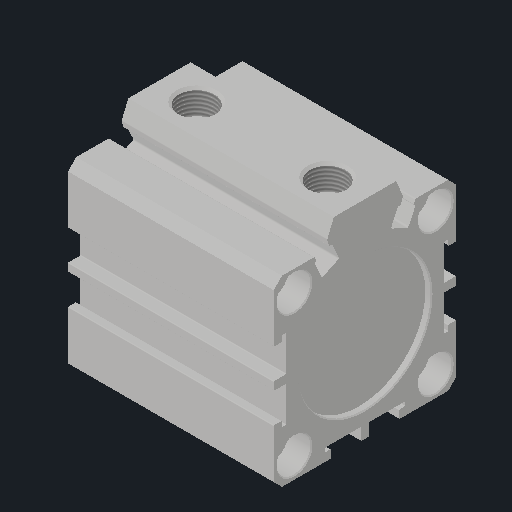
# Autodesk Inventor part: SDA-32x2525_b
Saved by Autodesk Inventor 2022 (Build 260153000, 153)
## iProperties
Created: 2022-09-20
Part Number: SDA-32x2525_b
Material: Generic
Catalog Web Link: www.cadenas.de
Description: SDA SSA STA  Series - Body-Body
Vendor: AIRTAC
Document SubType Name: Modeling
Designer: psAdmin
Manufacturer: AIRTAC
Mass: 56.8028 g
Surface Area: 257.905 cm^2
Volume: 56.8028 cm^3
Density: 1 g/cm^3
Appearance: PSOLRGB-175-175-175
Category: PARTsolutions
Company: AIRTAC
PSOL_IDENT_0: {$CADENAS_DATA/23d-libs/airtac/pneumatic_equipment/cylinders/compact_cylinder/sda_series/parts/sda_s
PSOL_IDENT_1: sa_sta_body.prj},222 {VTYP=3D},{NB=SDA-32x2525_b},{LINA=SDA-32x25},{NN=SDA SSA STA  Series - Body},{
PSOL_IDENT_2: DATE=27.08.2021 03:42:34},{GEOMDATE=22.01.2019 02:43:44},{VERSION=},{LINEID=50},{WBVAR=TYPE,STROKE,S
PSOL_IDENT_3: TROKE1,MAGNET},{WBNUMERIC=STROKE,STROKE1}  {NB=SDA-32x2525_b},{LINA=SDA-32x25},{KT=DUMMY},{BORE=32},
PSOL_IDENT_4: {TYPE=SDA},{STROKE=25},{STROKE1=25},{MAGNET=},{ST1=5,10,15,20,25,30,35,40,45,50,55,60,65,70,75,80,85
PSOL_IDENT_5: ,90,100,110,120,130,[5:100]},{ORDER=SDA-32x25},{A=31.5},{B1=7.0},{C=24.5},{D=50.0},{E=12},{F=4},{G=3
PSOL_IDENT_6: .0},{K1=M6×1.0},{L=22.0},{M=3},{N1=9.0},{N2=9.0},{O=PT1/8},{P1=4.6},{P2=M6×1.0},{P3=16},{P4=5.5},{P5=
PSOL_IDENT_7: 8.2},{R=6},{S=44.000},{T1=34.0},{U=2.0},{V=12},{W=10},{X=18.3},{Y=15},{TYPE1='SDA', 'SDA Type', 'SSA'
PSOL_IDENT_8: , 'SSA Type', 'STA', 'STA Type'},{X1=40.5},{ST2=25}
NB: SDA-32x2525_b
NN: SDA SSA STA  Series - Body
NT: Body
NBSYN: $ORDER.$STROKE._b
LINA: SDA-32x25
CATALOG: AirTAC
BORE: 32
TYPE: SDA Type
STROKE: 25
STROKE1: 25
MAGNET: Without cushion
A: 31.5
B1: 7
C: 24.5
D: 50
E: 12
F: 4
G: 3
K1: M6×1.0
L: 22
M: 3
N1: 9
N2: 9
O: PT1/8
P1: 4.6
P2: M6×1.0
P3: 16
P4: 5.5
P5: 8.2
R: 6
S: 44
T1: 34
U: 2
V: 12
W: 10
X: 18.3
Y: 15
SUPPLIER: AIRTAC
ARTICLENO: SDA-32x2525_b
BOMINFO: SDA-32x25
CREATOR: CADENAS GmbH
Title: SDA-32x25
Author: Cadenas PARTsolutions
Comments: Body
Autodesk Inventor part; units mm, degrees
sketch "Sketch_1" plane through (0, 0, 0) normal (1, 0, 0) x (0, 1, 0)
  line L0 (0.8, 22) -> (-0.8, 22)
  arc A0 (-0.8, 22) -> (-1, 21.8) centre (-0.8, 21.8) ccw
  line L1 (-1, 21.8) -> (-1, 19.2)
  arc A1 (-1.2, 19) -> (-1, 19.2) centre (-1.2, 19.2) ccw
  line L2 (-1.2, 19) -> (-9.4, 19)
  arc A2 (-9.6, 19.2) -> (-9.4, 19) centre (-9.4, 19.2) ccw
  line L3 (-9.6, 19.2) -> (-9.6, 19.8)
  arc A3 (-9.4, 20) -> (-9.6, 19.8) centre (-9.4, 19.8) ccw
  line L4 (-9.4, 20) -> (-8.4, 20)
  arc A4 (-8.4, 20) -> (-8.2, 20.2) centre (-8.4, 20.2) ccw
  line L5 (-8.2, 20.2) -> (-8.2, 21.8)
  arc A5 (-8.2, 21.8) -> (-8.4, 22) centre (-8.4, 21.8) ccw
  line L6 (-8.4, 22) -> (-20, 22)
  line L7 (-20, 22) -> (-22, 20)
  line L8 (-22, 20) -> (-22, 8.4)
  arc A6 (-22, 8.4) -> (-21.8, 8.2) centre (-21.8, 8.4) ccw
  line L9 (-21.8, 8.2) -> (-20.2, 8.2)
  arc A7 (-20.2, 8.2) -> (-20, 8.4) centre (-20.2, 8.4) ccw
  line L10 (-20, 8.4) -> (-20, 9.4)
  arc A8 (-19.8, 9.6) -> (-20, 9.4) centre (-19.8, 9.4) ccw
  line L11 (-19.8, 9.6) -> (-19.2, 9.6)
  arc A9 (-19, 9.4) -> (-19.2, 9.6) centre (-19.2, 9.4) ccw
  line L12 (-19, 9.4) -> (-19, 1.2)
  arc A10 (-19.2, 1) -> (-19, 1.2) centre (-19.2, 1.2) ccw
  line L13 (-19.2, 1) -> (-21.8, 1)
  arc A11 (-21.8, 1) -> (-22, 0.8) centre (-21.8, 0.8) ccw
  line L14 (-22, 0.8) -> (-22, -0.8)
  arc A12 (-22, -0.8) -> (-21.8, -1) centre (-21.8, -0.8) ccw
  line L15 (-21.8, -1) -> (-19.2, -1)
  arc A13 (-19, -1.2) -> (-19.2, -1) centre (-19.2, -1.2) ccw
  line L16 (-19, -1.2) -> (-19, -9.4)
  arc A14 (-19.2, -9.6) -> (-19, -9.4) centre (-19.2, -9.4) ccw
  line L17 (-19.2, -9.6) -> (-19.8, -9.6)
  arc A15 (-20, -9.4) -> (-19.8, -9.6) centre (-19.8, -9.4) ccw
  line L18 (-20, -9.4) -> (-20, -8.4)
  arc A16 (-20, -8.4) -> (-20.2, -8.2) centre (-20.2, -8.4) ccw
  line L19 (-20.2, -8.2) -> (-21.8, -8.2)
  arc A17 (-21.8, -8.2) -> (-22, -8.4) centre (-21.8, -8.4) ccw
  line L20 (-22, -8.4) -> (-22, -20)
  line L21 (-22, -20) -> (-20, -22)
  line L22 (-20, -22) -> (-8.4, -22)
  arc A18 (-8.4, -22) -> (-8.2, -21.8) centre (-8.4, -21.8) ccw
  line L23 (-8.2, -21.8) -> (-8.2, -20.2)
  arc A19 (-8.2, -20.2) -> (-8.4, -20) centre (-8.4, -20.2) ccw
  line L24 (-8.4, -20) -> (-9.4, -20)
  arc A20 (-9.6, -19.8) -> (-9.4, -20) centre (-9.4, -19.8) ccw
  line L25 (-9.6, -19.8) -> (-9.6, -19.2)
  arc A21 (-9.4, -19) -> (-9.6, -19.2) centre (-9.4, -19.2) ccw
  line L26 (-9.4, -19) -> (-1.2, -19)
  arc A22 (-1, -19.2) -> (-1.2, -19) centre (-1.2, -19.2) ccw
  line L27 (-1, -19.2) -> (-1, -21.8)
  arc A23 (-1, -21.8) -> (-0.8, -22) centre (-0.8, -21.8) ccw
  line L28 (-0.8, -22) -> (0.8, -22)
  arc A24 (0.8, -22) -> (1, -21.8) centre (0.8, -21.8) ccw
  line L29 (1, -21.8) -> (1, -19.2)
  arc A25 (1.2, -19) -> (1, -19.2) centre (1.2, -19.2) ccw
  line L30 (1.2, -19) -> (9.4, -19)
  arc A26 (9.6, -19.2) -> (9.4, -19) centre (9.4, -19.2) ccw
  line L31 (9.6, -19.2) -> (9.6, -19.8)
  arc A27 (9.4, -20) -> (9.6, -19.8) centre (9.4, -19.8) ccw
  line L32 (9.4, -20) -> (8.4, -20)
  arc A28 (8.4, -20) -> (8.2, -20.2) centre (8.4, -20.2) ccw
  line L33 (8.2, -20.2) -> (8.2, -21.8)
  arc A29 (8.2, -21.8) -> (8.4, -22) centre (8.4, -21.8) ccw
  line L34 (8.4, -22) -> (20, -22)
  line L35 (20, -22) -> (22, -20)
  line L36 (22, -20) -> (22, -12.3893)
  arc A30 (22, -12.3893) -> (21.769, -12.0268) centre (21.6, -12.3893) ccw
  line L37 (21.769, -12.0268) -> (21.1236, -11.7258)
  arc A31 (21.1236, -11.7258) -> (20.8578, -11.8226) centre (21.039, -11.9071) ccw
  line L38 (20.8578, -11.8226) -> (20.7733, -12.0038)
  arc A32 (20.5075, -12.1006) -> (20.7733, -12.0038) centre (20.592, -11.9193) ccw
  line L39 (20.5075, -12.1006) -> (17.1541, -10.5369)
  arc A33 (16.9607, -10.0053) -> (17.1541, -10.5369) centre (17.3232, -10.1744) ccw
  line L40 (16.9607, -10.0053) -> (18.5666, -6.5613)
  arc A34 (19.0982, -6.3679) -> (18.5666, -6.5613) centre (18.9291, -6.7304) ccw
  line L41 (19.0982, -6.3679) -> (22.4515, -7.9315)
  arc A35 (22.5483, -8.1973) -> (22.4515, -7.9315) centre (22.367, -8.1128) ccw
  line L42 (22.5483, -8.1973) -> (22.4749, -8.3546)
  arc A36 (22.4749, -8.3546) -> (22.5947, -8.6294) centre (22.6562, -8.4391) ccw
  line L43 (22.5947, -8.6294) -> (23.96, -9.0702)
  arc A37 (23.96, -9.0702) -> (24.2359, -9.0591) centre (24.0829, -8.6896) ccw
  line L44 (24.2359, -9.0591) -> (28, -7.5)
  line L45 (28, -7.5) -> (28, 7.5)
  line L46 (28, 7.5) -> (24.2359, 9.0591)
  arc A38 (24.2359, 9.0591) -> (23.96, 9.0702) centre (24.0829, 8.6896) ccw
  line L47 (23.96, 9.0702) -> (22.5947, 8.6294)
  arc A39 (22.5947, 8.6294) -> (22.4749, 8.3546) centre (22.6562, 8.4391) ccw
  line L48 (22.4749, 8.3546) -> (22.5483, 8.1973)
  arc A40 (22.4515, 7.9315) -> (22.5483, 8.1973) centre (22.367, 8.1128) ccw
  line L49 (22.4515, 7.9315) -> (19.0982, 6.3679)
  arc A41 (18.5666, 6.5613) -> (19.0982, 6.3679) centre (18.9291, 6.7304) ccw
  line L50 (18.5666, 6.5613) -> (16.9607, 10.0053)
  arc A42 (17.1541, 10.5369) -> (16.9607, 10.0053) centre (17.3232, 10.1744) ccw
  line L51 (17.1541, 10.5369) -> (20.5075, 12.1006)
  arc A43 (20.7733, 12.0038) -> (20.5075, 12.1006) centre (20.592, 11.9193) ccw
  line L52 (20.7733, 12.0038) -> (20.8578, 11.8226)
  arc A44 (20.8578, 11.8226) -> (21.1236, 11.7258) centre (21.039, 11.9071) ccw
  line L53 (21.1236, 11.7258) -> (21.769, 12.0268)
  arc A45 (21.769, 12.0268) -> (22, 12.3893) centre (21.6, 12.3893) ccw
  line L54 (22, 12.3893) -> (22, 20)
  line L55 (22, 20) -> (20, 22)
  line L56 (20, 22) -> (8.4, 22)
  arc A46 (8.4, 22) -> (8.2, 21.8) centre (8.4, 21.8) ccw
  line L57 (8.2, 21.8) -> (8.2, 20.2)
  arc A47 (8.2, 20.2) -> (8.4, 20) centre (8.4, 20.2) ccw
  line L58 (8.4, 20) -> (9.4, 20)
  arc A48 (9.6, 19.8) -> (9.4, 20) centre (9.4, 19.8) ccw
  line L59 (9.6, 19.8) -> (9.6, 19.2)
  arc A49 (9.4, 19) -> (9.6, 19.2) centre (9.4, 19.2) ccw
  line L60 (9.4, 19) -> (1.2, 19)
  arc A50 (1, 19.2) -> (1.2, 19) centre (1.2, 19.2) ccw
  line L61 (1, 19.2) -> (1, 21.8)
  arc A51 (1, 21.8) -> (0.8, 22) centre (0.8, 21.8) ccw
  constraints: 124 end point, 104 point on circle, 52 centre point
extrude "Extrusion1" add sketch "Sketch_1" along normal blind 49.5
sketch "Sketch_4" plane through (0, 0, 17) normal (0, 0, 1) x (1, 0, 0)
  line L0 (24.75, -17) -> (0, -17)
  line L1 (0, -17) -> (0, -12.65)
  line L2 (0, -12.65) -> (0.25, -12.9)
  line L3 (0.25, -12.9) -> (5.5, -12.9)
  line L4 (5.5, -12.9) -> (5.5, -14)
  line L5 (5.5, -14) -> (6.0415, -14.5415)
  line L6 (6.0415, -14.5415) -> (15.4585, -14.5415)
  line L7 (15.4585, -14.5415) -> (16, -14)
  line L8 (16, -14) -> (16, -14.7)
  line L9 (16, -14.7) -> (24.75, -14.7)
  line L10 (24.75, -14.7) -> (24.75, -17)
  line L11 (24.75, -17) -> (0, -17)
  constraints: 24 end point
revolve "Revolution1" cut sketch "Sketch_4" angle 360 about axis through (24.75, -17, 17) along (1, 0, 0)
thread "Thread1" size "M6x1" class "6H" standard "ISO Metric profile" full length
pattern_linear "Rectangular Pattern1" count 2 spacing 34 along (0, 0, -1) count 2 spacing 34 along (0, 1, 0) of "Revolution1"
sketch "Sketch_5" plane through (0, 0, 17) normal (0, 0, 1) x (1, 0, 0)
  line L0 (49.5, -17) -> (24.75, -17)
  line L1 (24.75, -17) -> (24.75, -14.7)
  line L2 (24.75, -14.7) -> (33.5, -14.7)
  line L3 (33.5, -14.7) -> (33.5, -14)
  line L4 (33.5, -14) -> (34.0415, -14.5415)
  line L5 (34.0415, -14.5415) -> (43.4585, -14.5415)
  line L6 (43.4585, -14.5415) -> (44, -14)
  line L7 (44, -14) -> (44, -12.9)
  line L8 (44, -12.9) -> (49.25, -12.9)
  line L9 (49.25, -12.9) -> (49.5, -12.65)
  line L10 (49.5, -12.65) -> (49.5, -17)
  line L11 (49.5, -17) -> (24.75, -17)
  constraints: 24 end point
revolve "Revolution2" cut sketch "Sketch_5" angle 360 about axis through (49.5, -17, 17) along (1, 0, 0)
thread "Thread2" size "M6x1" class "6H" standard "ISO Metric profile" full length
pattern_linear "Rectangular Pattern2" count 2 spacing 34 along (0, 0, -1) count 2 spacing 34 along (0, 1, 0) of "Revolution2"
sketch "Sketch4" plane through (0, 28, 7.5) normal (0, 1, 0) x (1, 0, 0)
  point P0 (9, 7.5)
hole "Hole1" at (9, 28, 0) direction (0, -1, 0) diameter 8.566 depth 6 countersink diameter 9.728 countersink angle 90 thread size "G9.728x0.907" designation "G 1/8" standard "ISO Pipe Threads"
sketch "Sketch5" plane through (0, 28, 7.5) normal (0, 1, 0) x (1, 0, 0)
  point P0 (40.5, 7.5)
hole "Hole2" at (40.5, 28, 0) direction (0, -1, 0) diameter 8.566 depth 6 countersink diameter 9.728 countersink angle 90 thread size "G9.728x0.907" designation "G 1/8" standard "ISO Pipe Threads"
sketch "Sketch_10" plane through (0, 0, 0) normal (0, 0, 1) x (1, 0, 0)
  line L0 (43.5, 0) -> (0, 0)
  line L1 (0, 0) -> (0, 6)
  line L2 (0, 6) -> (11.3, 6)
  line L3 (11.3, 6) -> (11.3, 16)
  line L4 (11.3, 16) -> (43.5, 16)
  line L5 (43.5, 16) -> (43.5, 0)
  line L6 (43.5, 0) -> (0, 0)
  constraints: 14 end point
revolve "Revolution3" cut sketch "Sketch_10" angle 360 about axis through (43.5, 0, 0) along (1, 0, 0)
sketch "Sketch_11" plane through (0, 0, 0) normal (0, 0, 1) x (1, 0, 0)
  line L0 (2.5, 0) -> (0, 0)
  line L1 (0, 0) -> (0, 17.4)
  line L2 (0, 17.4) -> (0.4, 17)
  line L3 (0.4, 17) -> (2.5, 17)
  line L4 (2.5, 17) -> (2.5, 0)
  line L5 (2.5, 0) -> (0, 0)
  constraints: 12 end point
revolve "Revolution4" cut sketch "Sketch_11" angle 360 about axis through (2.5, 0, 0) along (1, 0, 0)
sketch "Sketch_13" plane through (0, 0, 0) normal (0, 0, 1) x (1, 0, 0)
  line L0 (2.5, 0) -> (-3, 0)
  line L1 (-3, 6) -> (2.5, 6)
  line L2 (2.5, 6) -> (2.5, 11)
  line L3 (2.5, 11) -> (-2, 11)
  arc A0 (-2, 11) -> (-3, 10) centre (-2, 10) ccw
  line L4 (-3, 10) -> (-3, 6)
  constraints: 10 end point, 2 point on circle, 1 centre point
revolve "Revolution5" add sketch "Sketch_13" angle 360 about axis through (2.5, 0, 0) along (1, 0, 0)
sketch "Sketch9" plane through (49.5, 0, 0) normal (1, 0, 0) x (0, 0, -1)
  point P0 (0, 0)
hole "Hole3" at (49.5, 0, 0) direction (-1, 0, 0) diameter 32 depth 1.5 countersink diameter 32.5 countersink angle 90
ref_plane "IP_SWITCH1_XY" through (1, 17.7636, -8.2833) normal (-1, 0, 0) x (0, 0, -1)
ref_plane "IP_SWITCH1_YZ" through (1, 17.7636, -8.2833) normal (0, 0, -1) x (0, -1, 0)
ref_plane "IP_SWITCH1_ZX" through (1, 17.7636, -8.2833) normal (0, -1, 0) x (-1, 0, 0)
ref_plane "IP_SWITCH2_XY" through (48.5, 17.7636, 8.2833) normal (1, 0, 0) x (0, 0, -1)
ref_plane "IP_SWITCH2_YZ" through (48.5, 17.7636, 8.2833) normal (0, 0, -1) x (0, 1, 0)
ref_plane "IP_SWITCH2_ZX" through (48.5, 17.7636, 8.2833) normal (0, 1, 0) x (1, 0, 0)
ref_plane "IP_SWITCH3_XY" through (1, 1, -19) normal (-1, 0, 0) x (0, 0, -1)
ref_plane "IP_SWITCH3_YZ" through (1, 1, -19) normal (0, 0, -1) x (0, -1, 0)
ref_plane "IP_SWITCH3_ZX" through (1, 1, -19) normal (0, -1, 0) x (-1, 0, 0)
ref_plane "IP_SWITCH4_XY" through (48.5, -1, 19) normal (1, 0, 0) x (0, 0, -1)
ref_plane "IP_SWITCH4_YZ" through (48.5, -1, 19) normal (0, 0, -1) x (0, 1, 0)
ref_plane "IP_SWITCH4_ZX" through (48.5, -1, 19) normal (0, 1, 0) x (1, 0, 0)
ref_plane "for_dummy_XY" through (0, 0, 0) normal (-1, 0, 0) x (0, 0, -1)
ref_plane "for_dummy_YZ" through (0, 0, 0) normal (0, 0, -1) x (0, -1, 0)
ref_plane "for_dummy_ZX" through (0, 0, 0) normal (0, -1, 0) x (-1, 0, 0)
ref_plane "for_s_1_XY" through (9, 22, 0) normal (0, 1, 0) x (1, 0, 0)
ref_plane "for_s_1_YZ" through (9, 22, 0) normal (1, 0, 0) x (0, 0, -1)
ref_plane "for_s_1_ZX" through (9, 22, 0) normal (0, 0, -1) x (0, 1, 0)
ref_plane "for_s_2_XY" through (40.5, 22, 0) normal (0, 1, 0) x (1, 0, 0)
ref_plane "for_s_2_YZ" through (40.5, 22, 0) normal (1, 0, 0) x (0, 0, -1)
ref_plane "for_s_2_ZX" through (40.5, 22, 0) normal (0, 0, -1) x (0, 1, 0)
body "Solid1"
